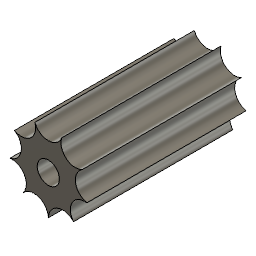
Reload Gear (Autodesk Fusion 360 design; units mm, degrees)
part number: 2026-08-23-16-41-29-549
Autodesk Fusion 360 part; units mm, degrees
note: some values were not read from the file. Set by a fixed rule: which sketch regions a step uses.
sketch "Sketch1" plane through (0, 0, 0) normal (0, 0, 1) x (1, 0, 0)
  line L0 (-6.1079, 16.7767) -> (-6.1049, 16.7778)
  line L1 (-15.4628, 8.9256) -> (-15.4612, 8.9284)
  line L2 (-17.5825, -3.1019) -> (-17.583, -3.0987)
  line L3 (-11.4751, -13.678) -> (-11.4776, -13.6759)
  line L4 (0.0016, -17.854) -> (-0.0016, -17.854)
  line L5 (11.4776, -13.6759) -> (11.4751, -13.678)
  line L6 (17.583, -3.0987) -> (17.5825, -3.1019)
  line L7 (15.4612, 8.9284) -> (15.4628, 8.9256)
  line L8 (6.1049, 16.7778) -> (6.1079, 16.7767)
  circle A0 centre (0, 0) radius 5
  arc A1 (-6.1079, 16.7767) -> (6.1079, 16.7767) centre (0, 19) ccw
  arc A2 (-15.4628, 8.9256) -> (-6.1049, 16.7778) centre (-12.213, 14.5548) ccw
  arc A3 (-17.5825, -3.1019) -> (-15.4612, 8.9284) centre (-18.7113, 3.2993) ccw
  arc A4 (-11.4751, -13.678) -> (-17.583, -3.0987) centre (-16.4545, -9.5) ccw
  arc A5 (0.0016, -17.854) -> (-11.4776, -13.6759) centre (-6.4984, -17.8542) ccw
  arc A6 (11.4776, -13.6759) -> (-0.0016, -17.854) centre (6.4984, -17.8542) ccw
  arc A7 (17.583, -3.0987) -> (11.4751, -13.678) centre (16.4545, -9.5) ccw
  arc A8 (15.4612, 8.9284) -> (17.5825, -3.1019) centre (18.7113, 3.2993) ccw
  arc A9 (6.1049, 16.7778) -> (15.4628, 8.9256) centre (12.213, 14.5548) ccw
  dimension "d1" = 19
  dimension "d2" = 10
  dimension "d3" = 13
  dimension "d5" = 360
  constraint coincident A0.centre origin
  measures "d1" distance of A0.centre A1.centre
  measures "d2" diameter of A0
  measures "d3" diameter of A1
extrude "Extrude1" add sketch "Sketch1" along normal blind 72 contours A1 A2 A3 A4 A5 A6 A7 A8 A9
